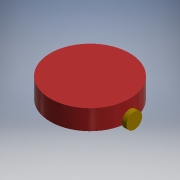
# Autodesk Inventor part: KobukiV3
Saved by Autodesk Inventor 2018 (Build 220112000, 112)
## iProperties
Part Number: KobukiV3
Material: Generic
Document SubType Name: Modeling
Designer: USER
Appearance: Generic
Author: USER
Autodesk Inventor part; units mm, degrees
ref_plane "YZ Plane" through (0, 0, 0) normal (1, 0, 0) x (0, 1, 0)
sketch "Sketch1" plane through (0, 0, 0) normal (0, 1, 0) x (-1, 0, 0)
  circle A0 centre (0, 0) radius 1770
  line L0 (-350, -1985) -> (350, -1985)
  line L1 (350, -1985) -> (350, -1775)
  line L2 (350, -1775) -> (-350, -1775)
  line L3 (-350, -1775) -> (-350, -1985)
  line L4 (-350, -1985) -> (350, -1775) construction
  line L5 (350, -1985) -> (-350, -1775) construction
  line L6 (-350, 1985) -> (350, 1985)
  line L7 (350, 1985) -> (350, 1775)
  line L8 (350, 1775) -> (-350, 1775)
  line L9 (-350, 1775) -> (-350, 1985)
  line L10 (-350, 1985) -> (350, 1775) construction
  line L11 (350, 1985) -> (-350, 1775) construction
  circle A1 centre (850, 0) radius 100
  point P0 (0, -1880)
  point P1 (0, 1880)
  dimension "d0" = 3540
  dimension "d1" = 700
  dimension "d2" = 210
  dimension "d3" = 700
  dimension "d4" = 210
  dimension "d5" = 200
  constraints: 24 end point, 4 midpoint, 4 parallel, 2 centre point, 2 horizontal, 2 perpendicular, 1 coincident
  measures "d0" diameter of A0
  measures "d1" distance of L2.end L1.end
  measures "d2" distance of L1.end L0.end
  measures "d3" distance of L7.end L8.end
  measures "d4" distance of L6.end L7.end
  measures "d5" diameter of A1
ref_plane "Work Plane1" through (0, 200, 0) normal (0, 1, 0) x (-1, 0, 0)
ref_plane "Work Plane2" through (0, 0, 1880) normal (0, 0, 1) x (1, 0, 0)
ref_plane "Work Plane3" through (0, 0, -1880) normal (0, 0, 1) x (1, 0, 0)
ref_plane "Work Plane4" through (0, 100, 0) normal (0, 1, 0) x (-1, 0, 0)
sketch "Sketch2" plane through (0, 200, 0) normal (0, 1, 0) x (-1, 0, 0)
  circle A0 centre (0, 0) radius 1770 projected
extrude "Extrusion1" add sketch "Sketch2" along normal blind 890
sketch "Sketch3" plane through (0, 0, 1880) normal (0, 0, 1) x (1, 0, 0)
  line L0 (350, 0) -> (-350, 0) projected
  circle A0 centre (0, 350) radius 350
  point P0 (0, 0)
  dimension "d12" = 700
  constraints: 1 centre point
  measures "d12" diameter of A0
extrude "Extrusion2" add sketch "Sketch3" along normal mid plane 210
sketch "Sketch4" plane through (0, 0, -1880) normal (0, 0, 1) x (1, 0, 0)
  circle A0 centre (0, 350) radius 350
  point P0 (0, 0)
  dimension "d15" = 700
  constraints: 1 centre point
  measures "d15" diameter of A0
extrude "Extrusion3" add sketch "Sketch4" along normal mid plane 210
sketch "Sketch5" plane through (0, 100, 0) normal (0, 1, 0) x (-1, 0, 0)
  circle A0 centre (850, 0) radius 100 projected
  circle A1 centre (850, 0) radius 100
  line L0 (950, 0) -> (750, 0)
  point P0 (0, 0)
  dimension "d18" = 200
  constraints: 2 end point, 2 point on circle, 1 centre point, 1 coincident, 1 concentric, 1 horizontal
  measures "d18" distance of L0.start L0.end
revolve "Revolution1" add sketch "Sketch5" angle 360 about axis through (-950, 100, 0) along (1, 0, 0) picked at (872.7518, -42.3477) contours A0 L0
body "Solid1"
